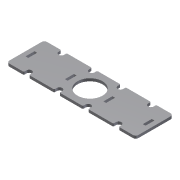
# Autodesk Inventor part: OpenROV_Dev_EChassis_Camera_Plate
Saved by Autodesk Inventor 2012 (Build 160160000, 160)
## iProperties
Created: 2012-08-08
Part Number: OpenROV_Dev_EChassis_Camera_Plate
Material: Default
Document SubType Name: Modeling
Designer: user
Density: 1 g/cm^3
Author: user
Autodesk Inventor part; units mm, degrees
ref_plane "YZ Plane" through (0, 0, 0) normal (1, 0, 0) x (0, 1, 0)
ref_plane "XZ Plane" through (0, 0, 0) normal (0, 1, 0) x (-1, 0, 0)
ref_plane "XY Plane" through (0, 0, 0) normal (0, 0, 1) x (1, 0, 0)
sketch "Sketch1" plane through (0, 0, 0) normal (0, 0, 1) x (1, 0, 0)
  line L0 (8, 26) -> (11, 26)
  line L1 (11, 26) -> (11, 16)
  line L2 (11, 16) -> (8, 16)
  circle A0 centre (75, 21) radius 14
  line L3 (8, 26) -> (8, 16)
  line L4 (3, 3) -> (3, 39)
  line L5 (52, 26) -> (55, 26)
  line L6 (55, 26) -> (55, 16)
  line L7 (55, 16) -> (52, 16)
  line L8 (52, 16) -> (52, 26)
  line L9 (95, 26) -> (98, 26)
  line L10 (98, 26) -> (98, 16)
  line L11 (98, 16) -> (95, 16)
  line L12 (95, 16) -> (95, 26)
  line L13 (147, 39) -> (147, 3)
  line L14 (142, 26) -> (139, 26)
  line L15 (139, 26) -> (139, 16)
  line L16 (139, 16) -> (142, 16)
  line L17 (142, 16) -> (142, 26)
  arc A1 (56, 39) -> (62, 39) centre (59, 39) ccw
  arc A2 (88, 39) -> (94, 39) centre (91, 39) ccw
  arc A3 (62, 3) -> (56, 3) centre (59, 3) ccw
  arc A4 (94, 3) -> (88, 3) centre (91, 3) ccw
  arc A5 (22, 39) -> (28, 39) centre (25, 39) ccw
  arc A6 (122, 39) -> (128, 39) centre (125, 39) ccw
  arc A7 (28, 3) -> (22, 3) centre (25, 3) ccw
  arc A8 (128, 3) -> (122, 3) centre (125, 3) ccw
  line L18 (22, 39) -> (22, 41)
  line L19 (28, 39) -> (28, 41)
  line L20 (122, 39) -> (122, 41)
  line L21 (128, 39) -> (128, 41)
  line L22 (128, 3) -> (128, 1)
  line L23 (122, 3) -> (122, 1)
  line L24 (22, 3) -> (22, 1)
  line L25 (28, 3) -> (28, 1)
  line L26 (6, 0) -> (21, 0)
  line L27 (129, 0) -> (144, 0)
  line L28 (129, 42) -> (144, 42)
  line L29 (6, 42) -> (21, 42)
  arc A9 (22, 41) -> (21, 42) centre (21, 41) ccw
  arc A10 (29, 42) -> (28, 41) centre (29, 41) ccw
  arc A11 (122, 41) -> (121, 42) centre (121, 41) ccw
  arc A12 (129, 42) -> (128, 41) centre (129, 41) ccw
  arc A13 (128, 1) -> (129, 0) centre (129, 1) ccw
  arc A14 (121, 0) -> (122, 1) centre (121, 1) ccw
  arc A15 (21, 0) -> (22, 1) centre (21, 1) ccw
  arc A16 (28, 1) -> (29, 0) centre (29, 1) ccw
  line L30 (56, 3) -> (56, 1)
  line L31 (62, 3) -> (62, 1)
  line L32 (88, 3) -> (88, 1)
  line L33 (94, 3) -> (94, 1)
  line L34 (94, 39) -> (94, 41)
  line L35 (88, 39) -> (88, 41)
  line L36 (56, 39) -> (56, 41)
  line L37 (62, 39) -> (62, 41)
  line L38 (29, 42) -> (55, 42)
  line L39 (63, 42) -> (87, 42)
  line L40 (95, 42) -> (121, 42)
  line L41 (95, 0) -> (121, 0)
  line L42 (29, 0) -> (55, 0)
  line L43 (63, 0) -> (87, 0)
  arc A17 (55, 0) -> (56, 1) centre (55, 1) ccw
  arc A18 (62, 1) -> (63, 0) centre (63, 1) ccw
  arc A19 (87, 0) -> (88, 1) centre (87, 1) ccw
  arc A20 (94, 1) -> (95, 0) centre (95, 1) ccw
  arc A21 (95, 42) -> (94, 41) centre (95, 41) ccw
  arc A22 (88, 41) -> (87, 42) centre (87, 41) ccw
  arc A23 (56, 41) -> (55, 42) centre (55, 41) ccw
  arc A24 (63, 42) -> (62, 41) centre (63, 41) ccw
  arc A25 (6, 42) -> (3, 39) centre (6, 39) ccw
  arc A26 (3, 3) -> (6, 0) centre (6, 3) ccw
  arc A27 (144, 0) -> (147, 3) centre (144, 3) ccw
  arc A28 (147, 39) -> (144, 42) centre (144, 39) ccw
  point P0 (0, 0)
  point P1 (147, 42)
  point P2 (147, 0)
  point P3 (3, 42)
  point P4 (3, 0)
  dimension "d0" = 10
  dimension "d7" = 28
  dimension "d13" = 72
  dimension "d16" = 5
  dimension "d17" = 3
  dimension "d18" = 3
  dimension "d19" = 10
  dimension "d20" = 3
  dimension "d21" = 10
  dimension "d22" = 20
  dimension "d23" = 20
  dimension "d28" = 5
  dimension "d29" = 3
  dimension "d30" = 10
  dimension "d43" = 6
  dimension "d45" = 6
  dimension "d47" = 16
  dimension "d48" = 16
  dimension "d53" = 6
  dimension "d55" = 100
  dimension "d56" = 50
  dimension "d57" = 1
  dimension "d58" = 42
  dimension "d61" = 16
  dimension "d62" = 16
  dimension "d67" = 1
  dimension "d68" = 144
  dimension "d69" = 50
  dimension "d70" = 3
  dimension "d71" = 3
  dimension "d72" = 3
  dimension "d73" = 3
  dimension "d74" = 3
  dimension "d75" = 3
  dimension "d76" = 3
  constraints: 88 end point, 79 tangent, 62 perpendicular, 56 point on circle, 29 centre point, 17 equal radius, 12 parallel, 8 point on line, 3 horizontal, 1 collinear
  measures "d0" distance between parallel lines of L2 L0
  measures "d7" diameter of A0
  measures "d13" distance from line of L4 A0.centre
  measures "d16" distance between parallel lines of L4 L3
  measures "d17" distance between parallel lines of L1 L3
  measures "d18" distance between parallel lines of L6 L8
  measures "d19" distance between parallel lines of L7 L5
  measures "d20" distance between parallel lines of L10 L12
  measures "d21" distance between parallel lines of L9 L11
  measures "d22" distance from line of A0.centre L6
  measures "d23" distance from line of A0.centre L12
  measures "d28" distance between parallel lines of L17 L13
  measures "d29" distance of L14.start L14.end
  measures "d30" distance of L14.end L15.end
  measures "d43" diameter of A1
  measures "d45" diameter of A2
  measures "d47" horizontal distance of A0.centre A2.centre
  measures "d48" horizontal distance of A1.centre A0.centre
  measures "d53" diameter of A5
  measures "d55" distance of A6.centre A5.centre
  measures "d56" horizontal distance of A0.centre A5.centre
  measures "d57" radius of A9
  measures "d58" distance between parallel lines of L26 L29
  measures "d61" horizontal distance of A0.centre A3.centre
  measures "d62" horizontal distance of A0.centre A4.centre
  measures "d67" radius of A17
  measures "d68" distance between parallel lines of L13 L4
  measures "d69" horizontal distance of A6.centre A0.centre
  measures "d70" radius of A25
  measures "d71" distance from line of A2.centre L39
  measures "d72" distance from line of A1.centre L38
  measures "d73" distance from line of L42 A3.centre
  measures "d74" radius of A3
  measures "d75" radius of A4
  measures "d76" distance from line of L43 A4.centre
extrude "Extrusion4" add sketch "Sketch1" along normal blind 3
body "Solid4"
